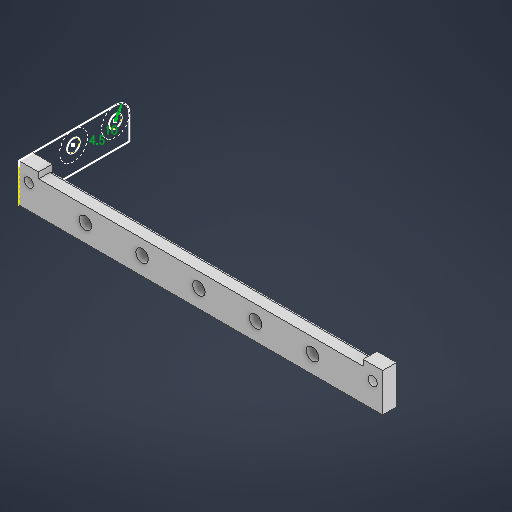
# Autodesk Inventor part: cpu_hold_plate
Saved by Autodesk Inventor 2026 (Build 300175000, 175)
## iProperties
Created: 2025-02-02
Part Number: cpu_hold_plate
Material: 一般
Document SubType Name: Modeling
Designer: nyxeon
Density: 1 g/cm^3
Appearance: 既定
Author: nyxeon
Autodesk Inventor part; units mm, degrees
ref_plane "YZ Plane" through (0, 0, 0) normal (1, 0, 0) x (0, 1, 0)
ref_plane "XZ Plane" through (0, 0, 0) normal (0, 1, 0) x (-1, 0, 0)
ref_plane "XY Plane" through (0, 0, 0) normal (0, 0, 1) x (1, 0, 0)
sketch "スケッチ1" plane through (0, 0, 0) normal (0, 0, 1) x (1, 0, 0)
  arc A0 (-17.9, -5.9192) -> (-17.6, -6.2192) centre (-17.6, -5.9192) ccw construction
  line L0 (-17.6, -6.2192) -> (-11.8244, -6.2192) construction
  line L1 (-11.8244, -6.2192) -> (-9.5, -2.219) projected
  arc A1 (-9.2172, -2.0192) -> (-9.5, -2.219) centre (-9.2172, -2.3192) ccw projected
  line L2 (-9.2172, -2.0192) -> (-6.9328, -2.0192) projected
  arc A2 (-6.65, -2.219) -> (-6.9328, -2.0192) centre (-6.9328, -2.3192) ccw projected
  line L3 (-6.65, -2.219) -> (-4.3256, -6.2192) projected
  line L4 (-4.3256, -6.2192) -> (8.4756, -6.2192) construction
  line L5 (8.4756, -6.2192) -> (10.8, -2.219) projected
  arc A3 (11.0828, -2.0192) -> (10.8, -2.219) centre (11.0828, -2.3192) ccw projected
  line L6 (11.0828, -2.0192) -> (13.3672, -2.0192) projected
  arc A4 (13.65, -2.219) -> (13.3672, -2.0192) centre (13.3672, -2.3192) ccw projected
  line L7 (13.65, -2.219) -> (15.9744, -6.2192) projected
  line L8 (15.9744, -6.2192) -> (21.25, -6.2192) construction
  arc A5 (21.25, -6.2192) -> (21.55, -5.9192) centre (21.25, -5.9192) ccw construction
  line L9 (21.55, -2.3692) -> (21.55, -5.9192) construction
  arc A6 (21.55, -2.3692) -> (21.25, -2.0692) centre (21.25, -2.3692) ccw construction
  line L10 (21.25, -2.0692) -> (17.65, -2.0692) construction
  arc A7 (17.65, 2.2308) -> (17.65, -2.0692) centre (17.65, 0.0808) ccw construction
  line L11 (17.65, 2.2308) -> (21.25, 2.2308) construction
  arc A8 (21.25, 2.2308) -> (21.55, 2.5308) centre (21.25, 2.5308) ccw construction
  line L12 (21.55, 4.8808) -> (21.55, 2.5308) construction
  line L13 (21.55, 4.8808) -> (-17.9, 4.8808) construction
  line L14 (-17.9, 4.8808) -> (-17.9, -5.9192) construction
  line L15 (1.3, 1.9308) -> (1.3, -1.7692) construction
  arc A9 (1, -2.0692) -> (1.3, -1.7692) centre (1, -1.7692) ccw construction
  line L16 (1, -2.0692) -> (-2.5, -2.0692) construction
  arc A10 (-2.5, 2.2308) -> (-2.5, -2.0692) centre (-2.5, 0.0808) ccw construction
  line L17 (-2.5, 2.2308) -> (1, 2.2308) construction
  arc A11 (1.3, 1.9308) -> (1, 2.2308) centre (1, 1.9308) ccw construction
  line L18 (-17.9, 5.3808) -> (21.55, 5.3808) construction
  circle A12 centre (-0.85, 0.0808) radius 2.15 construction
  line L19 (-0.85, 0.0808) -> (-2.5, 0.0808) construction
  circle A13 centre (-1.675, 0.0808) radius 2.25
  line L20 (64.025, 2.5048) -> (64.025, 91.3712) construction
  line L21 (-65.975, 91.3712) -> (-65.975, 2.5048) construction
  line L22 (64.025, 5.3808) -> (-65.975, 5.3808)
  circle A14 centre (18.625, 0.0808) radius 2.25
  circle A15 centre (38.925, 0.0808) radius 2.25
  circle A16 centre (59.225, 0.0808) radius 2.25
  circle A17 centre (-21.975, 0.0808) radius 2.25
  circle A18 centre (-1.675, 0.0808) radius 2.25
  circle A19 centre (18.625, 0.0808) radius 2.25
  circle A20 centre (38.925, 0.0808) radius 2.25
  circle A21 centre (-42.275, 0.0808) radius 2.25
  circle A22 centre (-21.975, 0.0808) radius 2.25
  circle A23 centre (-1.675, 0.0808) radius 2.25
  circle A24 centre (18.625, 0.0808) radius 2.25
  circle A25 centre (-62.575, 0.0808) radius 2.25
  circle A26 centre (-42.275, 0.0808) radius 2.25
  circle A27 centre (-21.975, 0.0808) radius 2.25
  circle A28 centre (-1.675, 0.0808) radius 2.25
  line L23 (64.025, 5.3808) -> (64.025, -6.2192)
  line L24 (64.025, -6.2192) -> (-65.975, -6.2192)
  line L25 (-65.975, -6.2192) -> (-65.975, 5.3808)
  point P0 (0, 0)
  dimension "d1" = 4.5
  dimension "d4" = 20.3
  dimension "d7" = 20.3
  constraints: 17 centre point, 10 end point, 5 point on line, 4 horizontal, 3 tangent, 1 collinear, 1 midpoint, 1 perpendicular, 30 other
  measures "d1" diameter of A13
  measures "d4" distance of A13.centre A14.centre
  measures "d7" distance of A13.centre A17.centre
extrude "押し出し1" add sketch "スケッチ1" along normal blind 5 contours L24 L25 L22 L23 L7 A4 L6 A3 L5 L3 A2 L2 A1 L1 | L1 A1 L2 A2 L3 L24 | L5 A3 L6 A4 L7 L24 | A16 | A25
sketch "スケッチ3" plane through (0, 0, 0) normal (0, 0, -1) x (-1, 0, 0)
  line L0 (9.5, -2.219) -> (11.8244, -6.2192) projected
  arc A0 (9.5, -2.219) -> (9.2172, -2.0192) centre (9.2172, -2.3192) ccw projected
  line L1 (6.9328, -2.0192) -> (9.2172, -2.0192) projected
  arc A1 (6.9328, -2.0192) -> (6.65, -2.219) centre (6.9328, -2.3192) ccw projected
  line L2 (4.3256, -6.2192) -> (6.65, -2.219) projected
  line L3 (65.975, -6.2192) -> (-64.025, -6.2192) projected
  point P0 (0, 0)
extrude "押し出し2" cut sketch "スケッチ3" against normal through all
pattern_linear "矩形状パターン1" count 4 spacing 20.3 along (1, 0, 0) count 3 spacing 20.3 along (-1, 0, 0) of "押し出し2"
sketch "スケッチ4" plane through (-65.975, -6.2192, 0) normal (-1, 0, 0) x (0, 0, 1)
  circle A0 centre (0.55, 8.724) radius 2.1 construction
  circle A1 centre (-14.45, 8.724) radius 2.1 construction
  circle A2 centre (-29.45, 8.724) radius 2.1 construction
  line L0 (0, 0) -> (5, 0) projected
  line L1 (5, 11.6) -> (5, 0) projected
  line L2 (0, 11.6) -> (5, 11.6) construction
  circle A3 centre (-29.45, 8.724) radius 5 construction
  circle A4 centre (-14.45, 8.724) radius 5 construction
  line L3 (0, 0) -> (5, 0) construction
  line L4 (0, 0) -> (-34.45, 0)
  line L5 (-34.45, 0) -> (-34.45, 8.724)
  line L6 (-29.45, 13.724) -> (-14.45, 13.724)
  line L7 (-14.45, 13.724) -> (5, 13.724)
  line L8 (5, 0) -> (5, 11.6) construction
  line L9 (5, 13.724) -> (5, 11.6)
  arc A5 (-29.45, 13.724) -> (-34.45, 8.724) centre (-29.45, 8.724) ccw
  circle A6 centre (-29.45, 8.724) radius 2.25
  circle A7 centre (-14.45, 8.724) radius 2.25
  circle A8 centre (0.55, 8.724) radius 2.25
  point P0 (0, 6.2192)
  dimension "d20" = 10
  dimension "d21" = 4.5
  constraints: 10 end point, 6 coincident, 5 centre point, 4 horizontal, 4 point on circle, 2 equal radius, 1 perpendicular, 1 tangent, 1 vertical, 1 vertical alignment, 3 other
  measures "d20" diameter of A3
  measures "d21" diameter of A6
sketch "スケッチ5" plane through (0, 0, 5) normal (0, 0, 1) x (1, 0, 0)
  line L0 (64.025, 5.3808) -> (-65.975, 5.3808) construction
  line L1 (64.025, -6.2192) -> (64.025, 5.3808) projected
  line L2 (64.025, 5.3808) -> (57.025, 5.3808)
  line L3 (57.025, 5.3808) -> (57.025, 7.5048)
  line L4 (57.025, 7.5048) -> (64.025, 7.5048)
  line L5 (64.025, 7.5048) -> (64.025, 5.3808)
  line L6 (-65.975, 5.3808) -> (-58.975, 5.3808)
  line L7 (-58.975, 5.3808) -> (-58.975, 7.5048)
  line L8 (-58.975, 7.5048) -> (-65.975, 7.5048)
  line L9 (-65.975, 7.5048) -> (-65.975, 5.3808)
  circle A0 centre (-42.275, 0.0808) radius 2.25 projected
  line L10 (-17.9, -5.9192) -> (-17.9, 4.8808) construction
  circle A1 centre (-1.675, 0.0808) radius 2.25 projected
  point P0 (0, 0)
  dimension "d22" = 11.6
  dimension "d23" = 2.124
  dimension "d24" = 7
  dimension "d30" = 16.7
  dimension "d31" = 16.225
  constraints: 16 end point, 4 parallel, 2 equal length, 2 horizontal, 2 perpendicular
  measures "d22" distance of L1.start L0.start
  measures "d23" distance between parallel lines of L4 L0
  measures "d24" distance of L3.end L4.end
  measures "d30" distance from line of L7 A0.centre
  measures "d31" distance from line of L10 A1.centre
extrude "押し出し3" add sketch "スケッチ5" against normal up to surface (5 mm away) contours L2 L3 L4 L5 | L9 L8 L7 L6
sketch "スケッチ6" plane through (0, 0, 0) normal (0, 0, -1) x (-1, 0, 0)
  line L0 (-57.025, 7.5048) -> (-64.025, 7.5048) construction
  line L1 (-64.025, -6.2192) -> (-64.025, 7.5048) construction
  circle A0 centre (-60.525, 2.5048) radius 1.65
  line L2 (-64.025, 7.5048) -> (-57.025, 7.5048) projected
  line L3 (65.975, 7.5048) -> (58.975, 7.5048) construction
  line L4 (65.975, -6.2192) -> (65.975, 7.5048) construction
  circle A1 centre (62.475, 2.5048) radius 1.65
  point P0 (0, 0)
  dimension "d32" = 3.3
  dimension "d33" = 3.5
  dimension "d34" = 5
  dimension "d35" = 3.5
  dimension "d36" = 5
  constraints: 2 centre point, 1 equal radius
  measures "d32" diameter of A0
  measures "d33" distance from line of A0.centre L1
  measures "d34" distance from line of L2 A0.centre
  measures "d35" distance from line of L4 A1.centre
  measures "d36" distance from line of A1.centre L3
extrude "押し出し4" cut sketch "スケッチ6" against normal through all
fillet "フィレット1" radius 1 1 edges at (-0.975, 5.3808, 0)
sketch "スケッチ7" plane through (0, 0, 5) normal (0, 0, 1) x (1, 0, 0)
  line L0 (-52.4244, -6.2192) -> (-50.1, -2.219) projected
  arc A0 (-49.8172, -2.0192) -> (-50.1, -2.219) centre (-49.8172, -2.3192) ccw projected
  line L1 (-49.8172, -2.0192) -> (-47.5328, -2.0192) projected
  arc A1 (-47.25, -2.219) -> (-47.5328, -2.0192) centre (-47.5328, -2.3192) ccw projected
  line L2 (-47.25, -2.219) -> (-44.9256, -6.2192) projected
  line L3 (-32.1244, -6.2192) -> (-29.8, -2.219) projected
  arc A2 (-29.5172, -2.0192) -> (-29.8, -2.219) centre (-29.5172, -2.3192) ccw projected
  line L4 (-29.5172, -2.0192) -> (-27.2328, -2.0192) projected
  arc A3 (-26.95, -2.219) -> (-27.2328, -2.0192) centre (-27.2328, -2.3192) ccw projected
  line L5 (-26.95, -2.219) -> (-24.6256, -6.2192) projected
  line L6 (-11.8244, -6.2192) -> (-9.5, -2.219) projected
  arc A4 (-9.2172, -2.0192) -> (-9.5, -2.219) centre (-9.2172, -2.3192) ccw projected
  line L7 (-9.2172, -2.0192) -> (-6.9328, -2.0192) projected
  arc A5 (-6.65, -2.219) -> (-6.9328, -2.0192) centre (-6.9328, -2.3192) ccw projected
  line L8 (-6.65, -2.219) -> (-4.3256, -6.2192) projected
  line L9 (8.4756, -6.2192) -> (10.8, -2.219) projected
  arc A6 (11.0828, -2.0192) -> (10.8, -2.219) centre (11.0828, -2.3192) ccw projected
  line L10 (11.0828, -2.0192) -> (13.3672, -2.0192) projected
  arc A7 (13.65, -2.219) -> (13.3672, -2.0192) centre (13.3672, -2.3192) ccw projected
  line L11 (13.65, -2.219) -> (15.9744, -6.2192) projected
  line L12 (28.7756, -6.2192) -> (31.1, -2.219) projected
  arc A8 (31.3828, -2.0192) -> (31.1, -2.219) centre (31.3828, -2.3192) ccw projected
  line L13 (31.3828, -2.0192) -> (33.6672, -2.0192) projected
  arc A9 (33.95, -2.219) -> (33.6672, -2.0192) centre (33.6672, -2.3192) ccw projected
  line L14 (33.95, -2.219) -> (36.2744, -6.2192) projected
  line L15 (49.0756, -6.2192) -> (51.4, -2.219) projected
  arc A10 (51.6828, -2.0192) -> (51.4, -2.219) centre (51.6828, -2.3192) ccw projected
  line L16 (51.6828, -2.0192) -> (53.9672, -2.0192) projected
  arc A11 (54.25, -2.219) -> (53.9672, -2.0192) centre (53.9672, -2.3192) ccw projected
  line L17 (54.25, -2.219) -> (56.5744, -6.2192) projected
  line L18 (-52.4244, -6.2192) -> (-44.9256, -6.2192)
  line L19 (-24.6256, -6.2192) -> (-26.95, -2.219) projected
  line L20 (-32.1244, -6.2192) -> (-24.6256, -6.2192)
  line L21 (-9.5, -2.219) -> (-11.8244, -6.2192) projected
  line L22 (-11.8244, -6.2192) -> (-4.3256, -6.2192)
  line L23 (15.9744, -6.2192) -> (8.4756, -6.2192)
  line L24 (36.2744, -6.2192) -> (33.95, -2.219) projected
  line L25 (28.7756, -6.2192) -> (36.2744, -6.2192)
  line L26 (49.0756, -6.2192) -> (56.5744, -6.2192)
  point P0 (0, 0)
  constraints: 12 end point, 4 horizontal
extrude "押し出し5" add sketch "スケッチ7" against normal blind 4
equation "\"d35\" = d33"
equation "\"d36\" = d34"
